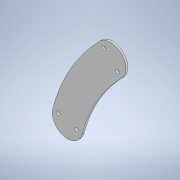
# Autodesk Inventor part: TurretHoodPanel3
Saved by Autodesk Inventor 2022 (Build 260153000, 153)
## iProperties
Created: 2022-01-18
Part Number: TurretHoodPanel3
Material: Generic
Document SubType Name: Modeling
Designer: tagaz
Density: 1 g/cm^3
Appearance: Default
Author: tagaz
Autodesk Inventor part; units mm, degrees
ref_plane "YZ Plane" through (0, 0, 0) normal (1, 0, 0) x (0, 1, 0)
ref_plane "XZ Plane" through (0, 0, 0) normal (0, 1, 0) x (-1, 0, 0)
ref_plane "XY Plane" through (0, 0, 0) normal (0, 0, 1) x (1, 0, 0)
sketch "Sketch1" plane through (0, 0, 0) normal (0, 0, 1) x (1, 0, 0)
  arc A0 (-197.5656, 197.5656) -> (-269.8797, 72.314) centre (0, 0) ccw construction
  arc A1 (-215.5261, 215.5261) -> (-294.4142, 78.888) centre (0, 0) ccw
  arc A2 (-179.6051, 179.6051) -> (-245.3452, 65.74) centre (0, 0) ccw
  arc A3 (-179.6051, 179.6051) -> (-215.5261, 215.5261) centre (-197.5656, 197.5656) ccw
  arc A4 (-294.4142, 78.888) -> (-245.3452, 65.74) centre (-269.8797, 72.314) ccw
  line L0 (0, 0) -> (-269.8797, 72.314) construction
  line L1 (0, 0) -> (269.8797, -72.314) construction
  line L2 (0, 0) -> (-197.5656, 197.5656) construction
  line L3 (0, 0) -> (-111.7396, 0) construction
  circle A5 centre (-208.791, 208.791) radius 3.175
  line L4 (-215.5261, 215.5261) -> (-179.6051, 179.6051) construction
  circle A6 centre (-285.2137, 76.4228) radius 3.175
  circle A7 centre (-254.5456, 68.2053) radius 3.175
  circle A8 centre (-186.3403, 186.3403) radius 3.175
  line L5 (-294.4142, 78.888) -> (-245.3452, 65.74) construction
  dimension "d30" = 279.4
  dimension "d31" = 180
  dimension "d32" = 30
  dimension "d33" = 50.8
  dimension "d34" = 45
  dimension "d35" = 6.35
  dimension "d36" = 15.875
  dimension "d37" = 6.35
  dimension "d38" = 6.35
  dimension "d39" = 6.35
  dimension "d40" = 15.875
  dimension "d41" = 15.875
  dimension "d42" = 15.875
  constraints: 12 end point, 10 point on circle, 9 centre point, 4 point on line, 4 tangent, 3 collinear, 1 coincident, 1 horizontal, 1 other
  measures "d30" radius of A0
  measures "d31" angle of L0 L1
  measures "d32" angle of L2 L0
  measures "d33" diameter of A3
  measures "d34" angle of L3 L2
  measures "d35" diameter of A5
  measures "d36" distance of L2.end A5.centre
  measures "d37" diameter of A6
  measures "d38" diameter of A7
  measures "d39" diameter of A8
  measures "d40" distance of L2.end A8.centre
  measures "d41" distance of L0.end A7.centre
  measures "d42" distance of L0.end A6.centre
extrude "Extrusion1" add sketch "Sketch1" along normal blind 3.175
body "Solid1"
